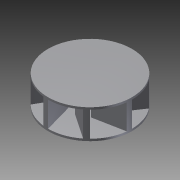
# Autodesk Inventor part: Box fan
Saved by Autodesk Inventor 2012 (Build 160160000, 160)
## iProperties
Created: 2011-08-19
Part Number: Box fan
Material: Default
Document SubType Name: Modeling
Designer: Minh Tran
Density: 1 g/cm^3
Author: Minh Tran
Autodesk Inventor part; units mm, degrees
ref_plane "YZ Plane" through (0, 0, 0) normal (1, 0, 0) x (0, 1, 0)
ref_plane "XZ Plane" through (0, 0, 0) normal (0, 1, 0) x (-1, 0, 0)
sketch "Sketch1" plane through (0, 0, 0) normal (0, 0, 1) x (1, 0, 0)
  circle A0 centre (0, 0) radius 50.8
  dimension "d0" = 101.6
  constraints: 1 centre point, 1 coincident
  measures "d0" diameter of A0
extrude "Extrusion1" add sketch "Sketch1" along normal blind 2.54
sketch "Sketch2" plane through (0, 0, 2.54) normal (0, 0, 1) x (1, 0, 0)
  circle A0 centre (0, 0) radius 50.8 projected
  arc A1 (5.858, 50.4611) -> (-0.0279, 50.8) centre (0, 0) ccw
  arc A2 (12.9209, 13.9983) -> (9.6237, 16.4404) centre (0, 0) ccw
  line L0 (-0.0279, 50.8) -> (9.6237, 16.4404)
  line L1 (5.858, 50.4611) -> (12.9209, 13.9983)
  arc A3 (39.8236, 31.5392) -> (35.9013, 35.9408) centre (0, 0) ccw
  arc A4 (19.0348, 0.7618) -> (18.4301, 4.8202) centre (0, 0) ccw
  line L2 (35.9013, 35.9408) -> (18.4301, 4.8202)
  line L3 (39.8236, 31.5392) -> (19.0348, 0.7618)
  arc A5 (50.4611, -5.858) -> (50.8, 0.0279) centre (0, 0) ccw
  arc A6 (13.9983, -12.9209) -> (16.4404, -9.6237) centre (0, 0) ccw
  line L4 (50.8, 0.0279) -> (16.4404, -9.6237)
  line L5 (50.4611, -5.858) -> (13.9983, -12.9209)
  arc A7 (31.5392, -39.8236) -> (35.9408, -35.9013) centre (0, 0) ccw
  arc A8 (0.7618, -19.0348) -> (4.8202, -18.4301) centre (0, 0) ccw
  line L6 (35.9408, -35.9013) -> (4.8202, -18.4301)
  line L7 (31.5392, -39.8236) -> (0.7618, -19.0348)
  arc A9 (-5.858, -50.4611) -> (0.0279, -50.8) centre (0, 0) ccw
  arc A10 (-12.9209, -13.9983) -> (-9.6237, -16.4404) centre (0, 0) ccw
  line L8 (0.0279, -50.8) -> (-9.6237, -16.4404)
  line L9 (-5.858, -50.4611) -> (-12.9209, -13.9983)
  arc A11 (-39.8236, -31.5392) -> (-35.9013, -35.9408) centre (0, 0) ccw
  arc A12 (-19.0348, -0.7618) -> (-18.4301, -4.8202) centre (0, 0) ccw
  line L10 (-35.9013, -35.9408) -> (-18.4301, -4.8202)
  line L11 (-39.8236, -31.5392) -> (-19.0348, -0.7618)
  arc A13 (-50.4611, 5.858) -> (-50.8, -0.0279) centre (0, 0) ccw
  arc A14 (-13.9983, 12.9209) -> (-16.4404, 9.6237) centre (0, 0) ccw
  line L12 (-50.8, -0.0279) -> (-16.4404, 9.6237)
  line L13 (-50.4611, 5.858) -> (-13.9983, 12.9209)
  arc A15 (-31.5392, 39.8236) -> (-35.9408, 35.9013) centre (0, 0) ccw
  arc A16 (-0.7618, 19.0348) -> (-4.8202, 18.4301) centre (0, 0) ccw
  line L14 (-35.9408, 35.9013) -> (-4.8202, 18.4301)
  line L15 (-31.5392, 39.8236) -> (-0.7618, 19.0348)
  dimension "d7" = 360
  constraints: 34 point on circle, 32 end point, 16 centre point, 10 coincident, 81 other
extrude "Extrusion2" add sketch "Sketch2" along normal blind 30.48 contours A0 L5 A6 L4 | L3 A4 L2 A0 | A0 L7 A8 L6 | L1 A2 L0 A0 | A0 L9 A10 L8 | L15 A16 L14 A0 | A0 L11 A12 L10 | L13 A14 L12 A0
ref_plane "Work Plane1" through (0, 0, 35.56) normal (0, 0, 1) x (1, 0, 0)
sketch "Sketch3" plane through (0, 0, 35.56) normal (0, 0, 1) x (1, 0, 0)
  circle A0 centre (0, 0) radius 50.8
  dimension "d12" = 101.6
  constraints: 1 centre point, 1 coincident
  measures "d12" diameter of A0
extrude "Extrusion3" add sketch "Sketch3" against normal blind 2.54
body "Solid1"
